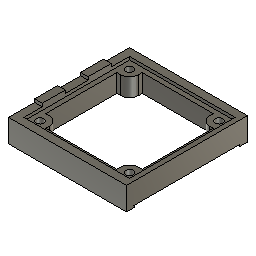
frame control adapter (Autodesk Fusion 360 design; units mm, degrees)
Autodesk Fusion 360 part; units mm, degrees
sketch "Skizze1" plane through (0, 0, 0) normal (0, 0, 1) x (1, 0, 0)
  line L0 (19.25, -19.75) -> (-19.25, -19.75)
  line L1 (-19.25, -19.75) -> (-19.25, 19.75)
  line L2 (-19.25, 19.75) -> (19.25, 19.75)
  line L3 (19.25, 19.75) -> (19.25, -19.75)
  line L4 (19.25, -19.75) -> (-19.25, 19.75) construction
  line L5 (-19.25, -19.75) -> (19.25, 19.75) construction
  dimension "d1" = 38.5
  dimension "d2" = 39.5
  constraint horizontal L0
  constraint perpendicular L0 L1
  constraint parallel L0 L2
  constraint parallel L1 L3
  constraint coincident L4 origin
  constraint coincident L5 origin
  measures "d1" distance of L1.end L2.end
  measures "d2" distance of L0.end L1.end
extrude "Extrusion1" add sketch "Skizze1" along normal blind 7.5
sketch "Skizze2" plane through (0, 0, 7.5) normal (0, 0, 1) x (-1, 0, 0)
  line L0 (-19.25, -19.75) -> (19.25, -19.75)
  line L1 (19.25, -19.75) -> (19.25, 19.75)
  line L2 (19.25, 19.75) -> (-19.25, 19.75)
  line L3 (-19.25, 19.75) -> (-19.25, -19.75)
  line L4 (16.75, 17.25) -> (-17.75, 17.25)
  line L5 (-17.75, 17.25) -> (-17.75, -17.25)
  line L6 (-17.75, -17.25) -> (16.75, -17.25)
  line L7 (16.75, -17.25) -> (16.75, 17.25)
  dimension "d5" = 2.5
  dimension "d6" = 2.5
  dimension "d7" = 2.5
  constraint horizontal L4
  constraint vertical L5
  constraint horizontal L6
  constraint vertical L7
  constraint equal L6 L7
  measures "d5" distance of L1 L7
  measures "d6" distance of L2 L4
  measures "d7" distance of L0 L6
extrude "Extrusion2" cut sketch "Skizze2" against normal blind 1 contours L4 L5 L6 L7
sketch "Skizze3" plane through (0, 0, 0) normal (0, 0, -1) x (1, 0, 0)
  line L0 (-19.25, -19.75) -> (19.25, -19.75)
  line L1 (19.25, -19.75) -> (19.25, 19.75)
  line L2 (19.25, 19.75) -> (-19.25, 19.75)
  line L3 (-19.25, 19.75) -> (-19.25, -19.75)
  line L4 (-16.75, -17.25) -> (17.75, -17.25)
  line L5 (-16.75, 17.25) -> (-16.75, -17.25)
  line L6 (17.75, 17.25) -> (-16.75, 17.25)
  line L7 (17.75, -17.25) -> (17.75, 17.25)
extrude "Extrusion3" cut sketch "Skizze3" against normal blind 0.6 contours L4 L5 L6 L7
sketch "Skizze4" plane through (0, 0, 6.5) normal (0, 0, 1) x (-1, 0, 0)
  line L0 (16.75, -17.25) -> (16.75, 17.25)
  line L1 (16.75, 17.25) -> (-17.75, 17.25)
  line L2 (-17.75, 17.25) -> (-17.75, -17.25)
  line L3 (-17.75, -17.25) -> (16.75, -17.25)
  line L4 (15.25, -15.75) -> (-16.25, -15.75)
  line L5 (-16.25, -15.75) -> (-16.25, 15.75)
  line L6 (-16.25, 15.75) -> (15.25, 15.75)
  line L7 (15.25, 15.75) -> (15.25, -15.75)
  line L8 (14.105, -14.605) -> (-15.105, -14.605) construction
  line L9 (-15.105, -14.605) -> (-15.105, 14.605) construction
  line L10 (-15.105, 14.605) -> (14.105, 14.605) construction
  line L11 (14.105, 14.605) -> (14.105, -14.605) construction
  line L12 (14.105, -14.605) -> (16.75, -17.25) construction
  line L13 (14.105, 14.605) -> (16.75, 17.25) construction
  line L14 (14.105, -11.605) -> (15.25, -11.605)
  line L15 (11.105, -14.605) -> (11.105, -15.75)
  line L16 (-12.105, -14.605) -> (-12.105, -15.75)
  line L17 (-15.105, -11.605) -> (-16.25, -11.605)
  line L18 (-15.105, 11.605) -> (-16.25, 11.605)
  line L19 (-12.105, 14.605) -> (-12.105, 15.75)
  line L20 (14.105, 11.605) -> (15.25, 11.605)
  line L21 (11.105, 14.605) -> (11.105, 15.75)
  arc A0 (11.105, 14.605) -> (14.105, 11.605) centre (14.105, 14.605) ccw
  arc A1 (14.105, -11.605) -> (11.105, -14.605) centre (14.105, -14.605) ccw
  arc A2 (-12.105, -14.605) -> (-15.105, -11.605) centre (-15.105, -14.605) ccw
  arc A3 (-15.105, 11.605) -> (-12.105, 14.605) centre (-15.105, 14.605) ccw
  dimension "d12" = 1.5
  dimension "d13" = 1.5
  dimension "d14" = 1.5
  dimension "d15" = 1.5
  dimension "d16" = 6
  dimension "d17" = 29.21
  constraint horizontal L4
  constraint vertical L5
  constraint horizontal L6
  constraint vertical L7
  constraint horizontal L8
  constraint vertical L9
  constraint horizontal L10
  constraint vertical L11
  constraint coincident L9.end L10.start
  constraint coincident L8.start L11.end
  constraint coincident L8.end L9.start
  constraint coincident L10.end L11.start
  constraint equal L8 L11
  constraint coincident L0.start L3.end
  constraint coincident L0.end L1.start
  constraint perpendicular L12 L13
  constraint equal L12 L13
  constraint equal A1 A2
  constraint equal A0 A3
  constraint equal A0 A1
  constraint coincident L11 L14.start
  constraint coincident L7 L14.end
  constraint tangent L14 A1
  constraint coincident L8 L15.start
  constraint coincident L4 L15.end
  constraint tangent L15 A1
  constraint coincident L8 L16.start
  constraint coincident L4 L16.end
  constraint tangent L16 A2
  constraint coincident L9 L17.start
  constraint coincident L5 L17.end
  constraint tangent L17 A2
  constraint coincident L9 L18.start
  constraint coincident L5 L18.end
  constraint tangent L18 A3
  constraint coincident L10 L19.start
  constraint coincident L6 L19.end
  constraint tangent L19 A3
  constraint coincident L11 L20.start
  constraint coincident L7 L20.end
  constraint tangent L20 A0
  constraint coincident L10 L21.start
  constraint coincident L6 L21.end
  constraint tangent L21 A0
  measures "d12" distance of L0 L7
  measures "d13" distance of L3 L4
  measures "d14" distance of L1 L6
  measures "d15" distance of L2 L5
  measures "d16" diameter of A1
  measures "d17" distance of L8.start L10.end
extrude "Extrusion4" cut sketch "Skizze4" against normal through all contours L4 L5 L6 L7 L14 L15 L16 L17 L18 L19 L20 L21 A0 A1 A2 A3
sketch "Skizze5" plane through (0, 0, 6.5) normal (0, 0, 1) x (-1, 0, 0)
  line L0 (-12.105, 15.75) -> (11.105, 15.75)
  line L1 (11.105, 15.75) -> (11.105, 14.605)
  arc A0 (11.105, 14.605) -> (14.105, 11.605) centre (14.105, 14.605) ccw
  line L2 (14.105, 11.605) -> (15.25, 11.605)
  line L3 (15.25, 11.605) -> (15.25, -11.605)
  line L4 (15.25, -11.605) -> (14.105, -11.605)
  arc A1 (14.105, -11.605) -> (11.105, -14.605) centre (14.105, -14.605) ccw
  line L5 (11.105, -14.605) -> (11.105, -15.75)
  line L6 (11.105, -15.75) -> (-12.105, -15.75)
  line L7 (-12.105, -15.75) -> (-12.105, -14.605)
  arc A2 (-12.105, -14.605) -> (-15.105, -11.605) centre (-15.105, -14.605) ccw
  line L8 (-15.105, -11.605) -> (-16.25, -11.605)
  line L9 (-16.25, -11.605) -> (-16.25, 11.605)
  line L10 (-16.25, 11.605) -> (-15.105, 11.605)
  arc A3 (-15.105, 11.605) -> (-12.105, 14.605) centre (-15.105, 14.605) ccw
  line L11 (-12.105, 14.605) -> (-12.105, 15.75)
  line L12 (16.75, -17.25) -> (16.75, 17.25)
  line L13 (16.75, 17.25) -> (-17.75, 17.25)
  line L14 (-17.75, 17.25) -> (-17.75, -17.25)
  line L15 (-17.75, -17.25) -> (16.75, -17.25)
  circle A4 centre (14.105, -14.605) radius 1.25
  circle A5 centre (14.105, 14.605) radius 1.25
  circle A6 centre (-15.105, -14.605) radius 1.25
  circle A7 centre (-15.105, 14.605) radius 1.25
  dimension "d19" = 2.5
  constraint concentric A1 A4
  constraint concentric A0 A5
  constraint concentric A2 A6
  constraint concentric A3 A7
  constraint equal A4 A6
  constraint equal A4 A5
  constraint equal A4 A7
  measures "d19" diameter of A4
extrude "Extrusion5" cut sketch "Skizze5" against normal through all contours A4 | A5 | A6 | A7
sketch "Skizze6" plane through (0, 0, 7.5) normal (0, 0, 1) x (-1, 0, 0)
  line L0 (-17.75, 17.25) -> (16.75, 17.25)
  line L1 (16.75, 17.25) -> (16.75, -17.25)
  line L2 (16.75, -17.25) -> (-17.75, -17.25)
  line L3 (-17.75, -17.25) -> (-17.75, 17.25)
  line L4 (-19.25, -19.75) -> (19.25, -19.75)
  line L5 (19.25, -19.75) -> (19.25, 19.75)
  line L6 (19.25, 19.75) -> (-19.25, 19.75)
  line L7 (-19.25, 19.75) -> (-19.25, -19.75)
  line L8 (16.75, -11.25) -> (19.25, -11.25)
  line L9 (19.25, -11.25) -> (19.25, -3.75)
  line L10 (19.25, -3.75) -> (16.75, -3.75)
  line L11 (16.75, -3.75) -> (16.75, -11.25)
  line L12 (16.75, 3.75) -> (19.25, 3.75)
  line L13 (19.25, 3.75) -> (19.25, 11.25)
  line L14 (19.25, 11.25) -> (16.75, 11.25)
  line L15 (16.75, 11.25) -> (16.75, 3.75)
  line L16 (19.25, -3.75) -> (19.25, 3.75) construction
  dimension "d21" = 7.5
  dimension "d22" = 15
  constraint horizontal L8
  constraint vertical L9
  constraint horizontal L10
  constraint vertical L11
  constraint coincident L5 L9.end
  constraint coincident L1 L8.start
  constraint horizontal L12
  constraint vertical L13
  constraint horizontal L14
  constraint vertical L15
  constraint coincident L5 L13.end
  constraint coincident L1 L12.start
  constraint midpoint L5 L16
  constraint equal L9 L13
  measures "d21" distance of L12.end L13.end
  measures "d22" distance of L8 L12
extrude "Extrusion6" add sketch "Skizze6" along normal blind 1 contours L1 L5 L12 L13 L14 L15 | L1 L5 L8 L9 L10 L11
sketch "Skizze7" plane through (0, 0, 0) normal (0, 0, -1) x (1, 0, 0)
  line L0 (-16.75, 17.25) -> (17.75, 17.25)
  line L1 (17.75, 17.25) -> (17.75, -17.25)
  line L2 (17.75, -17.25) -> (-16.75, -17.25)
  line L3 (-16.75, -17.25) -> (-16.75, 17.25)
  line L4 (-19.25, -19.75) -> (19.25, -19.75)
  line L5 (19.25, -19.75) -> (19.25, 19.75)
  line L6 (19.25, 19.75) -> (-19.25, 19.75)
  line L7 (-19.25, 19.75) -> (-19.25, -19.75)
  line L8 (17.75, 17.25) -> (19.25, 17.25)
  line L9 (19.25, 17.25) -> (19.25, -17.25)
  line L10 (19.25, -17.25) -> (17.75, -17.25)
  line L11 (17.75, -17.25) -> (17.75, 17.25)
  constraint horizontal L8
  constraint vertical L9
  constraint horizontal L10
  constraint vertical L11
  constraint coincident L5 L9.end
  constraint coincident L0.end L1.start
  constraint coincident L1.end L2.start
extrude "Extrusion7" cut sketch "Skizze7" against normal up to surface (0.6 mm away) contours L1 L5 L8 L9 L10 L11
equation "d7 = d6"
equation "d13 = d12"
equation "d14 = d12"
equation "d15 = d12"
